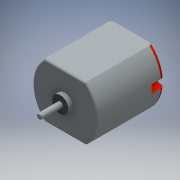
# Autodesk Inventor part: motorcito
Saved by Autodesk Inventor 2016 (Build 200138000, 138)
## iProperties
Created: 2018-01-03
Part Number: motorcito
Material: Genérico
Document SubType Name: Sheet Metal
Designer: David
Density: 1 g/cm^3
Sheet Metal Rule: Por defecto_mm
Appearance: Valor por defecto
Author: David
Autodesk Inventor part; units mm, degrees
ref_plane "YZ Plane" through (0, 0, 0) normal (1, 0, 0) x (0, 1, 0)
ref_plane "XZ Plane" through (0, 0, 0) normal (0, 1, 0) x (-1, 0, 0)
ref_plane "XY Plane" through (0, 0, 0) normal (0, 0, 1) x (1, 0, 0)
sketch "Boceto1" plane through (0, 0, 0) normal (0, 1, 0) x (-1, 0, 0)
  line L0 (0, 0) -> (15, 0)
  line L1 (15, 20) -> (0, 20)
  arc A0 (15, 0) -> (15, 20) centre (5.8364, 10) ccw
  arc A1 (0, 20) -> (0, 0) centre (9.1636, 10) ccw
  constraints: 4 end point, 4 point on circle, 2 centre point, 1 horizontal, 1 parallel
extrude "Extrusión1" add sketch "Boceto1" along normal blind 20
sketch "Boceto3" plane through (0, 20, 0) normal (0, 1, 0) x (1, 0, 0)
  arc A0 (2.8056, -8.5) -> (2.8056, -11.5) centre (2.8056, -10) ccw
  line L0 (2.8056, -8.5) -> (4.3168, -8.5)
  line L1 (2.8056, -11.5) -> (4.3168, -11.5)
  arc A1 (0, -20) -> (4.3168, -11.5) centre (-9.1636, -10) ccw
  arc A2 (4.3168, -8.5) -> (0, 0) centre (-9.1636, -10) ccw
  line L2 (0, 0) -> (-7.5, 0)
  line L3 (0, -20) -> (-7.5, -20)
  line L4 (-7.5, -20) -> (-7.5, 0)
  constraints: 10 end point, 6 point on circle, 3 centre point, 2 horizontal
extrude "Extrusión2" add sketch "Boceto3" along normal blind 4.8
mirror "Simetría1" about plane through (-7.5, 20, 0) normal (-1, 0, 0) of "Extrusión2"
sketch "Boceto6" plane through (0, 0, 0) normal (0, 0, -1) x (-1, 0, 0)
  line L0 (15, 24.8) -> (19.3168, 24.8) projected
  line L1 (0, 0) -> (0, 24.8) projected
  line L2 (2, 20) -> (13, 20)
  line L3 (15, 0) -> (15, 24.8) projected
  line L4 (-1.3056, 20) -> (-2.8056, 20) projected
  line L5 (2, 20) -> (2, 23)
  line L6 (13, 20) -> (13, 23)
  line L7 (2, 23) -> (13, 23)
  constraints: 8 end point, 1 collinear, 1 horizontal, 1 perpendicular, 1 vertical
extrude "Extrusión3" add sketch "Boceto6" along normal blind 1.6
sketch "Boceto7" plane through (0, 24.8, 0) normal (0, 1, 0) x (1, 0, 0)
  line L0 (0, -20) -> (-15, -20) projected
  arc A0 (2.8056, -8.5) -> (2.8056, -11.5) centre (2.8056, -10) ccw projected
  arc A1 (-4.7896, -14.1728) -> (-10.2987, -14.1728) centre (-7.5441, -10) ccw
  line L1 (-4.7896, -14.1728) -> (-10.2987, -14.1728)
  circle A2 centre (-7.5441, -10) radius 1
  point P0 (0, 0)
  constraints: 2 centre point, 2 end point, 2 point on circle, 1 coincident, 1 horizontal
extrude "Extrusión4" add sketch "Boceto7" along normal blind 2.4
sketch "Boceto8" plane through (-7.5441, 24.8, 10) normal (0, 1, 0) x (1, 0, 0)
  circle A0 centre (0, 0) radius 0.9601
  point P0 (7.5441, 10)
  constraints: 1 centre point
extrude "Extrusión5" add sketch "Boceto8" along normal blind 3.1
sketch "Boceto9" plane through (0, 0, 0) normal (0, -1, 0) x (1, 0, 0)
  line L0 (0, 0) -> (-15, 0) projected
  line L1 (-15, 20) -> (0, 20) projected
  line L2 (0, 0) -> (0, 20)
  arc A0 (-15, 20) -> (-15, 0) centre (-5.8364, 10) ccw projected
  line L3 (-15, 20) -> (-15, 0)
  circle A1 centre (-7.5441, 10) radius 0.9601 projected
  circle A2 centre (-7.5441, 10) radius 3
  circle A3 centre (-7.5441, 10) radius 1
  constraints: 4 end point, 2 centre point, 2 coincident, 2 perpendicular
extrude "Extrusión6" add sketch "Boceto9" along normal blind 1.6 contours A2
sketch "Boceto10" plane through (-7.5441, 0, 10) normal (0, -1, 0) x (1, 0, 0)
  circle A0 centre (0, 0) radius 0.9912
  point P0 (7.5441, -10)
  constraints: 1 centre point
extrude "Extrusión7" add sketch "Boceto10" along normal blind 9.4
fillet "Empalme1" radius 0.4 1 edges at (-8.5353, -9.4, 10)
fillet "Empalme2" radius 0.4 1 edges at (-8.5043, 27.9, 10)
fillet "Empalme3" radius 0.7 4 edges at (-7.5, 0, 0) (4.4, 0, 10) (-19.4, 0, 10) (-7.5, 0, 20)
fillet "Empalme4" radius 1.3 4 edges at (-17.9298, 24.8, 3.8582) (-17.9298, 24.8, 16.1418) (2.9298, 24.8, 16.1418) (2.9298, 24.8, 3.8582)
fillet "Empalme5" radius 0.4 16 edges at (-14.2879, 24.501, 20) (-15, 12.1, 20) (-14.9184, 0.2013, 19.7912) (-0.7121, 24.501, 20) (0, 10.35, 20) (0, 21.75, 20) (-0.0816, 0.2013, 19.7912) (-7.5, 24.8, 20) (-14.2879, 24.501, 0) (-7.5, 24.8, 0) (-0.7121, 24.501, 0) (0, 10.35, 0) (0, 21.75, 0) (-0.0816, 0.2013, 0.2088) (-14.9184, 0.2013, 0.2088) (-15, 12.1, 0)
equation "\"Radio_pliegue\" = Grosor"
equation "\"Anchura_desahogo_plegado\" = Grosor"
equation "\"Profundidad_desahogo_plegado\" = 0.5 * Grosor"
equation "\"Tamaño_destalonado\" = 4 * Grosor"
equation "\"Remanente_mínimo\" = 2 * Grosor"
equation "\"Radiodetransición\" = Radio_pliegue"
equation "\"Tamaño_de_radio_de_Jacobi\" = Radio_pliegue"
equation "\"TamañoSeparación\" = Grosor"
equation "\"Grosor\" = 0.5"
